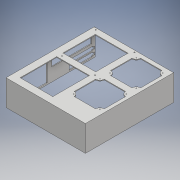
# Autodesk Inventor part: BackPlate
Saved by Autodesk Inventor 2017 (Build 210142000, 142)
## iProperties
Created: 2019-06-18
Part Number: BackPlate
Material: Generic
Document SubType Name: Modeling
Designer: DDeGo
Density: 1 g/cm^3
Appearance: Default
Author: DDeGo
Autodesk Inventor part; units mm, degrees
ref_plane "YZ Plane" through (0, 0, 0) normal (1, 0, 0) x (0, 1, 0)
ref_plane "XZ Plane" through (0, 0, 0) normal (0, 1, 0) x (-1, 0, 0)
ref_plane "XY Plane" through (0, 0, 0) normal (0, 0, 1) x (1, 0, 0)
sketch "Sketch1" plane through (0, 0, 0) normal (1, 0, 0) x (0, 1, 0)
  line L0 (0, 0) -> (350, 0)
  line L1 (350, 0) -> (350, 100)
  line L2 (350, 100) -> (0, 100)
  line L3 (0, 100) -> (0, 0)
  dimension "d0" = 100
  dimension "d1" = 350
  constraints: 8 end point, 2 parallel, 1 horizontal, 1 perpendicular
  measures "d0" distance between parallel lines of L0 L2
  measures "d1" distance between parallel lines of L3 L1
extrude "Extrusion1" add sketch "Sketch1" along normal blind 3
sketch "Sketch2" plane through (3, 0, 0) normal (1, 0, 0) x (0, 0, -1)
  line L0 (-97, 335) -> (-52.3, 335)
  line L1 (-52.3, 335) -> (-52.3, 176)
  line L2 (-52.3, 176) -> (-97, 176)
  line L3 (-97, 176) -> (-97, 335)
  line L4 (-6, 337.1) -> (-6, 245.9)
  line L5 (-6, 245.9) -> (-21.9, 245.9)
  line L6 (-21.9, 245.9) -> (-21.9, 337.1)
  line L7 (-18.7, 339.6) -> (-18.7, 347)
  line L8 (-18.7, 347) -> (-9.2, 347)
  line L9 (-9.2, 347) -> (-9.2, 339.6)
  line L10 (-19.4, 339.6) -> (-18.7, 339.6)
  line L11 (-9.2, 339.6) -> (-8.5, 339.6)
  arc A0 (-19.4, 339.6) -> (-21.9, 337.1) centre (-19.4, 337.1) ccw
  arc A1 (-6, 337.1) -> (-8.5, 339.6) centre (-8.5, 337.1) ccw
  line L12 (-93.9818, 5.5526) -> (-5.9818, 5.5526)
  line L13 (-5.9818, 5.5526) -> (-5.9818, 157.5526)
  line L14 (-5.9818, 157.5526) -> (-93.9818, 157.5526)
  line L15 (-93.9818, 157.5526) -> (-93.9818, 5.5526)
  line L16 (-26.175, 337.1) -> (-26.175, 245.9)
  line L17 (-26.175, 245.9) -> (-42.075, 245.9)
  line L18 (-42.075, 245.9) -> (-42.075, 337.1)
  line L19 (-38.875, 339.6) -> (-38.875, 347)
  line L20 (-38.875, 347) -> (-29.375, 347)
  line L21 (-29.375, 347) -> (-29.375, 339.6)
  line L22 (-39.575, 339.6) -> (-38.875, 339.6)
  line L23 (-29.375, 339.6) -> (-28.675, 339.6)
  arc A2 (-39.575, 339.6) -> (-42.075, 337.1) centre (-39.575, 337.1) ccw
  arc A3 (-26.175, 337.1) -> (-28.675, 339.6) centre (-28.675, 337.1) ccw
  line L24 (0, 350) -> (-100, 350) projected
  line L25 (0, 0) -> (0, 350) projected
  line L26 (-100, 350) -> (-100, 0) projected
  point P0 (-55.4956, 335.3765)
  dimension "d4" = 2.5
  dimension "d5" = 9.5
  dimension "d6" = 15.9
  dimension "d7" = 93.7
  dimension "d8" = 101.1
  dimension "d9" = 44.7
  dimension "d10" = 159
  dimension "d11" = 88
  dimension "d12" = 152
  dimension "d15" = 2.5
  dimension "d16" = 9.5
  dimension "d17" = 15.9
  dimension "d18" = 93.7
  dimension "d19" = 101.1
  dimension "d21" = 3
  dimension "d22" = 6
  dimension "d23" = 15
  dimension "d24" = 3
  dimension "d25" = 20.175
  constraints: 48 end point, 12 parallel, 8 point on circle, 8 tangent, 6 horizontal, 6 perpendicular, 5 collinear, 4 centre point, 2 equal radius, 2 vertical
  measures "d4" radius of A0
  measures "d5" distance between parallel lines of L9 L7
  measures "d6" distance between parallel lines of L6 L4
  measures "d7" distance from line of L5 L11.end
  measures "d8" distance between parallel lines of L5 L8
  measures "d9" distance of L0.start L0.end
  measures "d10" distance of L0.end L1.end
  measures "d11" distance of L12.start L12.end
  measures "d12" distance of L12.end L13.end
  measures "d15" radius of A2
  measures "d16" distance between parallel lines of L21 L19
  measures "d17" distance between parallel lines of L18 L16
  measures "d18" distance from line of L17 L23.end
  measures "d19" distance between parallel lines of L17 L20
  measures "d21" distance between parallel lines of L24 L8
  measures "d22" distance between parallel lines of L25 L4
  measures "d23" distance between parallel lines of L24 L0
  measures "d24" distance between parallel lines of L26 L3
  measures "d25" distance between parallel lines of L19 L7
extrude "Extrusion2" cut sketch "Sketch2" against normal through all
sketch "Sketch3" plane through (0, 0, 100) normal (0, 0, 1) x (1, 0, 0)
  line L0 (0, 0) -> (315, 0)
  line L1 (315, 0) -> (315, 350)
  line L2 (0, 350) -> (3, 350) projected
  line L3 (315, 350) -> (3, 350)
  line L4 (3, 350) -> (0, 350)
  line L5 (3, 0) -> (3, 350) projected
  line L6 (0, 350) -> (3, 350)
  line L7 (0, 350) -> (0, 0)
  dimension "d26" = 315
  constraints: 12 end point, 2 collinear, 2 horizontal, 2 perpendicular
  measures "d26" distance between parallel lines of L1 L7
extrude "Extrusion3" add sketch "Sketch3" along normal blind 3
sketch "Sketch4" plane through (3, 0, 100) normal (0, -1, 0) x (1, 0, 0)
  line L0 (312, 0) -> (312, 3) projected
  line L1 (-3, -100) -> (312, -100)
  line L2 (312, -100) -> (312, 3)
  line L3 (312, 3) -> (-3, 3)
  line L4 (-3, 3) -> (-3, -100)
  constraints: 8 end point, 2 parallel, 1 horizontal, 1 perpendicular
extrude "Extrusion4" add sketch "Sketch4" along normal blind 3
sketch "Sketch5" plane through (0, 0, 100) normal (0, 0, -1) x (-1, 0, 0)
  line L0 (-168.44, 341) -> (-13.5, 341) construction
  line L1 (-13.5, 341) -> (-13.5, 183.52) construction
  line L2 (-13.5, 183.52) -> (-168.44, 183.52) construction
  line L3 (-168.44, 183.52) -> (-168.44, 341) construction
  circle A0 centre (-13.5, 341) radius 2
  circle A1 centre (-168.44, 341) radius 2
  circle A2 centre (-168.44, 183.52) radius 2
  circle A3 centre (-36.36, 183.52) radius 2
  line L4 (-3, 0) -> (-3, 350) projected
  line L5 (-315, 350) -> (-3, 350) projected
  point P0 (0, 0)
  dimension "d31" = 157.48
  dimension "d32" = 154.94
  dimension "d33" = 22.86
  dimension "d34" = 4
  dimension "d35" = 10.5
  dimension "d36" = 9
  constraints: 8 end point, 4 centre point, 3 coincident, 3 equal radius, 2 parallel, 1 horizontal, 1 perpendicular, 1 point on line
  measures "d31" distance between parallel lines of L2 L0
  measures "d32" distance between parallel lines of L3 L1
  measures "d33" distance of L1.end A3.centre
  measures "d34" diameter of A1
  measures "d35" distance between parallel lines of L4 L1
  measures "d36" distance between parallel lines of L5 L0
extrude "Extrusion5" cut sketch "Sketch5" against normal through all
sketch "Sketch6" plane through (0, 0, 100) normal (0, 0, -1) x (-1, 0, 0)
  line L0 (-303.44, 333) -> (-183.44, 333)
  line L1 (-183.44, 333) -> (-183.44, 213)
  line L2 (-183.44, 213) -> (-303.44, 213)
  line L3 (-303.44, 213) -> (-303.44, 333)
  line L4 (-190.94, 325.5) -> (-295.94, 325.5) construction
  line L5 (-295.94, 325.5) -> (-295.94, 220.5) construction
  line L6 (-295.94, 220.5) -> (-190.94, 220.5) construction
  line L7 (-190.94, 220.5) -> (-190.94, 325.5) construction
  circle A0 centre (-295.94, 325.5) radius 1.5
  circle A1 centre (-190.94, 325.5) radius 1.5
  circle A2 centre (-190.94, 220.5) radius 1.5
  circle A3 centre (-295.94, 220.5) radius 1.5
  arc A4 (-303.44, 315.5) -> (-285.94, 333) centre (-303.44, 333) ccw
  arc A5 (-200.94, 333) -> (-183.44, 315.5) centre (-183.44, 333) ccw
  arc A6 (-183.44, 230.5) -> (-200.94, 213) centre (-183.44, 213) ccw
  arc A7 (-285.94, 213) -> (-303.44, 230.5) centre (-303.44, 213) ccw
  circle A8 centre (-168.44, 341) radius 2 projected
  line L8 (-315, 350) -> (-3, 350) projected
  line L9 (-303.44, 188) -> (-183.44, 188)
  line L10 (-183.44, 188) -> (-183.44, 68)
  line L11 (-183.44, 68) -> (-303.44, 68)
  line L12 (-303.44, 68) -> (-303.44, 188)
  line L13 (-190.94, 180.5) -> (-295.94, 180.5) construction
  line L14 (-295.94, 180.5) -> (-295.94, 75.5) construction
  line L15 (-295.94, 75.5) -> (-190.94, 75.5) construction
  line L16 (-190.94, 75.5) -> (-190.94, 180.5) construction
  circle A9 centre (-295.94, 180.5) radius 1.5
  circle A10 centre (-190.94, 180.5) radius 1.5
  circle A11 centre (-190.94, 75.5) radius 1.5
  circle A12 centre (-295.94, 75.5) radius 1.5
  arc A13 (-303.44, 170.5) -> (-285.94, 188) centre (-303.44, 188) ccw
  arc A14 (-200.94, 188) -> (-183.44, 170.5) centre (-183.44, 188) ccw
  arc A15 (-183.44, 85.5) -> (-200.94, 68) centre (-183.44, 68) ccw
  arc A16 (-285.94, 68) -> (-303.44, 85.5) centre (-303.44, 68) ccw
  line L17 (0, -3) -> (0, 350) projected
  point P0 (0, 0)
  point P1 (-329, 351)
  dimension "d39" = 105
  dimension "d40" = 120
  dimension "d41" = 105
  dimension "d42" = 3
  dimension "d43" = 35
  dimension "d46" = 15
  dimension "d47" = 17
  dimension "d48" = 105
  dimension "d49" = 120
  dimension "d50" = 105
  dimension "d51" = 3
  dimension "d52" = 35
  dimension "d53" = 25
  dimension "d63" = 183.44
  dimension "d64" = 265
  constraints: 32 end point, 16 centre point, 16 coincident, 16 point on circle, 16 point on line, 12 equal radius, 8 parallel, 4 perpendicular, 2 horizontal, 1 collinear, 6 other
  measures "d39" distance of L4.start L4.end
  measures "d40" distance of L0.start L0.end
  measures "d41" distance of L6.end L4.start
  measures "d42" diameter of A0
  measures "d43" diameter of A4
  measures "d46" distance from line of A8.centre L1
  measures "d47" distance between parallel lines of L8 L0
  measures "d48" distance of L16.end L14.start
  measures "d49" distance of L12.end L10.start
  measures "d50" distance of L15.end L16.end
  measures "d51" diameter of A9
  measures "d52" diameter of A13
  measures "d53" distance between parallel lines of L2 L9
  measures "d63" distance between parallel lines of L17 L1
  measures "d64" distance between parallel lines of L0 L11
extrude "Extrusion6" cut sketch "Sketch6" against normal through all contours L0 A5 L1 A6 L2 A7 L3 A4 | A0 | A1 | A2 | A3 | L9 A14 L10 A15 L11 A16 L12 A13 | A9 | A10 | A11 | A12
sketch "Sketch7" plane through (0, 0, 100) normal (0, 0, -1) x (-1, 0, 0)
  line L0 (-28, 325) -> (-158.44, 325)
  line L1 (-158.44, 325) -> (-158.44, 196.02)
  line L2 (-158.44, 196.02) -> (-28, 196.02)
  line L3 (-28, 196.02) -> (-28, 325)
  line L4 (-158.44, 171.02) -> (-28, 171.02)
  line L5 (-28, 171.02) -> (-28, 25)
  line L6 (-28, 25) -> (-158.44, 25)
  line L7 (-158.44, 25) -> (-158.44, 171.02)
  line L8 (-3, 0) -> (-3, 350) projected
  line L9 (-183.44, 315.5) -> (-183.44, 230.5) projected
  line L10 (-183.44, 170.5) -> (-183.44, 85.5) projected
  line L11 (-315, 350) -> (-3, 350) projected
  circle A0 centre (-36.36, 183.52) radius 2 projected
  line L12 (-3, 0) -> (-315, 0) projected
  point P0 (0, 0)
  dimension "d54" = 25
  dimension "d55" = 25
  dimension "d56" = 25
  dimension "d57" = 25
  dimension "d58" = 25
  dimension "d59" = 12.5
  dimension "d60" = 25
  constraints: 16 end point, 4 parallel, 2 horizontal, 2 perpendicular, 1 point on line
  measures "d54" distance between parallel lines of L5 L8
  measures "d55" distance between parallel lines of L9 L1
  measures "d56" distance between parallel lines of L10 L7
  measures "d57" distance between parallel lines of L2 L4
  measures "d58" distance between parallel lines of L11 L0
  measures "d59" distance from line of L2 A0.centre
  measures "d60" distance between parallel lines of L12 L6
extrude "Extrusion7" cut sketch "Sketch7" against normal through all contours L3 L2 L1 L0 | L4 L5 L6 L7
sketch "Sketch8" plane through (3, 350, 100) normal (0, 1, 0) x (1, 0, 0)
  line L0 (0, 100) -> (0, 0) projected
  line L1 (312, 0) -> (312, -3) projected
  line L2 (0, 0) -> (312, 0)
  line L3 (312, 0) -> (312, -3)
  line L4 (312, -3) -> (0, -3)
  line L5 (0, -3) -> (0, 0)
  point P0 (-3, 100)
  constraints: 8 end point, 2 parallel, 1 horizontal, 1 perpendicular
extrude "Extrusion8" cut sketch "Sketch8" against normal blind 1.5
fillet "Fillet1" radius 1.5 2 edges at (1.5, 350, 103) (1.5, 350, 0)
sketch "Sketch9" plane through (315, 0, 100) normal (1, 0, 0) x (0, 0, -1)
  line L0 (-3, -3) -> (100, -3) projected
  line L1 (-3, -3) -> (100, -3)
  line L2 (100, -3) -> (100, 348.5)
  line L3 (98.5, 350) -> (-1.5, 350)
  line L4 (-3, 348.5) -> (-3, -3)
  line L5 (98.5, 350) -> (-1.5, 350) projected
  line L6 (100, 0) -> (100, 348.5) projected
  arc A0 (100, 348.5) -> (98.5, 350) centre (98.5, 348.5) ccw projected
  arc A1 (-1.5, 350) -> (-3, 348.5) centre (-1.5, 348.5) ccw projected
  constraints: 8 end point, 4 point on circle, 2 collinear, 2 parallel, 1 horizontal, 1 perpendicular
extrude "Extrusion9" add sketch "Sketch9" along normal blind 1.5
body "Solid1"
